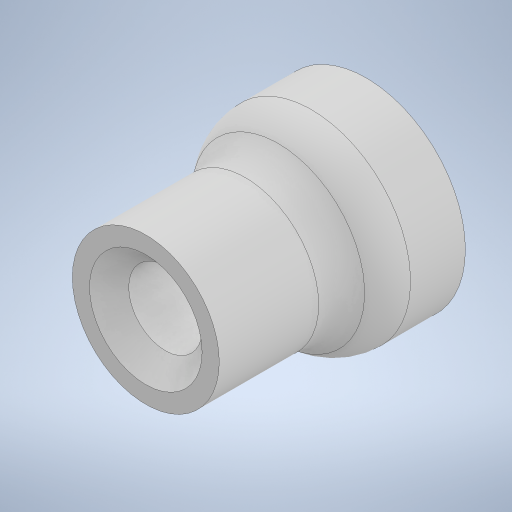
# Autodesk Inventor part: MagnetHolder
Saved by Autodesk Inventor 2024 (Build 280153000, 153)
## iProperties
Created: 2025-05-18
Part Number: MagnetHolder
Material: Ogólny
Document SubType Name: Modeling
Designer: Victoria
Density: 1 g/cm^3
Appearance: Domyślna
Author: Victoria
Autodesk Inventor part; units mm, degrees
ref_plane "YZ Plane" through (0, 0, 0) normal (1, 0, 0) x (0, 1, 0)
ref_plane "XZ Plane" through (0, 0, 0) normal (0, 1, 0) x (-1, 0, 0)
ref_plane "XY Plane" through (0, 0, 0) normal (0, 0, 1) x (1, 0, 0)
sketch "Szkic1" plane through (0, 0, 0) normal (0, 0, 1) x (1, 0, 0)
  circle A0 centre (0, 0) radius 2.55
  circle A1 centre (0, 0) radius 4.05
  dimension "d0" = 5.1
  dimension "d1" = 1.5
  constraints: 2 centre point, 1 coincident
  measures "d0" diameter of A0
  measures "d1" radial gap between concentric circles of A0 A1
extrude "Wyciągnięcie proste1" add sketch "Szkic1" along normal blind 3
sketch "Szkic2" plane through (0, 0, 3) normal (0, 0, 1) x (1, 0, 0)
  circle A0 centre (0, 0) radius 4.05 projected
  circle A1 centre (0, 0) radius 2.55 projected
extrude "Wyciągnięcie proste2" add sketch "Szkic2" along normal blind 1 contours A0 | A1
sketch "Szkic3" plane through (0, 0, 4) normal (0, 0, 1) x (1, 0, 0)
  circle A0 centre (0, 0) radius 1.5
  circle A1 centre (0, 0) radius 3
  dimension "d6" = 3
  dimension "d7" = 6
  constraints: 2 centre point, 2 coincident
  measures "d6" diameter of A0
  measures "d7" diameter of A1
extrude "Wyciągnięcie proste3" add sketch "Szkic3" along normal blind 5
fillet "Zaokrąglenie1" radius 2 2 edges at (-4.05, 0, 4) (-3, 0, 4)
chamfer "Faza1" distance 0.8 angle 45 1 edges at (-1.5, 0, 9)
chamfer "Faza2" distance 0.35 angle 45 1 edges at (-2.55, 0, 0)
